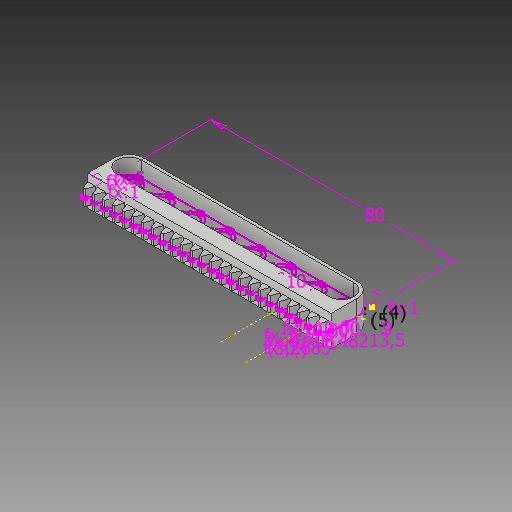
# Autodesk Inventor part: Gear_rack_8
Saved by Autodesk Inventor 2019 (Build 230136000, 136)
## iProperties
Created: 2019-01-28
Part Number: Gear_rack_8
Material: Generic
Document SubType Name: Modeling
Designer: Varga Daniel
Density: 1 g/cm^3
Appearance: Default
Author: Varga Daniel
Autodesk Inventor part; units mm, degrees
ref_plane "YZ Plane" through (0, 0, 0) normal (1, 0, 0) x (0, 1, 0)
ref_plane "XZ Plane" through (0, 0, 0) normal (0, 1, 0) x (-1, 0, 0)
ref_plane "XY Plane" through (0, 0, 0) normal (0, 0, 1) x (1, 0, 0)
derived "Base_part.ipt"
sketch "Sketch1" plane through (0, 0, 0) normal (0, 1, 0) x (-1, 0, 0)
  line L0 (5, 0) -> (25, 0)
  line L1 (30, 5) -> (30, 25)
  line L2 (25, 30) -> (5, 30)
  line L3 (0, 25) -> (0, 5)
  line L4 (5, 29) -> (25, 29)
  line L5 (29, 25) -> (29, 5)
  line L6 (25, 1) -> (5, 1)
  line L7 (1, 5) -> (1, 25)
  circle A0 centre (5, 5) radius 2.5
  circle A1 centre (5, 5) radius 3.5
  arc A2 (25, 0) -> (30, 5) centre (25, 5) ccw
  arc A3 (30, 25) -> (25, 30) centre (25, 25) ccw
  arc A4 (5, 30) -> (0, 25) centre (5, 25) ccw
  arc A5 (0, 5) -> (5, 0) centre (5, 5) ccw
  arc A6 (1, 5) -> (5, 1) centre (5, 5) ccw
  arc A7 (5, 29) -> (1, 25) centre (5, 25) ccw
  arc A8 (29, 25) -> (25, 29) centre (25, 25) ccw
  arc A9 (25, 1) -> (29, 5) centre (25, 5) ccw
  line L8 (49.1041, 15) -> (-27.081, 15) construction
  circle A10 centre (15, 5) radius 2.5
  circle A11 centre (15, 5) radius 3.5
  line L9 (31.1478, 10) -> (-2.4877, 10) construction
  line L10 (-2.8604, 5) -> (35.495, 5) construction
  line L11 (11.5359, 5.5) -> (8.4641, 5.5)
  line L12 (11.5359, 4.5) -> (8.4641, 4.5)
  line L13 (5, -2.5736) -> (5, 36.7522) construction
  line L14 (5.5, 1.5359) -> (5.5, 1)
  line L15 (4.5, 1.5359) -> (4.5, 1.0314)
  line L16 (28.9686, 4.5) -> (1.0314, 4.5)
  line L17 (29, 5.5) -> (1, 5.5)
  line L18 (15, -1.4978) -> (15, 34.8784) construction
  line L19 (15.5, 1.5359) -> (15.5, 1)
  line L20 (14.5, 1.5359) -> (14.5, 1)
  line L21 (1.5359, 5.5) -> (1, 5.5)
  line L22 (1.5359, 4.5) -> (1.0314, 4.5)
  line L23 (28.9686, 4.5) -> (8.4641, 4.5)
  line L24 (29, 5.5) -> (8.4641, 5.5)
  line L25 (4.5, 1.5359) -> (4.5, 1.0314)
  line L26 (5.5, 1.5359) -> (5.5, 1)
  line L27 (29, 10.5) -> (1, 10.5)
  line L28 (29, 9.5) -> (1, 9.5)
  line L29 (4.5, 28.9686) -> (4.5, 10.5)
  line L30 (4.5, 9.5) -> (4.5, 8.4641)
  line L31 (5.5, 29) -> (5.5, 10.5)
  line L32 (5.5, 9.5) -> (5.5, 8.4641)
  point P0 (0, 0)
  point P1 (30, 30)
  point P2 (0, 30)
  point P3 (5, 25)
sketch "Sketch2" plane through (0, 0, 0) normal (0, 1, 0) x (-1, 0, 0)
  circle A0 centre (15, 5) radius 3.5 construction
  circle A1 centre (15, 5) radius 2.5 construction
  line L0 (15.5, 1.5359) -> (15.5, 1) construction
  line L1 (14.5, 1.5359) -> (14.5, 1) construction
  line L2 (25, 1) -> (5, 1) construction
  line L3 (5, 0) -> (25, 0) construction
  arc A2 (0, 5) -> (5, 0) centre (5, 5) ccw construction
  arc A3 (1, 5) -> (5, 1) centre (5, 5) ccw construction
  circle A4 centre (5, 5) radius 3.5 construction
  circle A5 centre (5, 5) radius 2.5 construction
  line L4 (5, -2.5736) -> (5, 36.7522) construction
  line L5 (-2.8604, 5) -> (35.495, 5) construction
  line L6 (29, 5.5) -> (1, 5.5) construction
  line L7 (11.5359, 5.5) -> (8.4641, 5.5) construction
  line L8 (11.5359, 4.5) -> (8.4641, 4.5) construction
  line L9 (5.5, 1.5359) -> (5.5, 1) construction
  line L10 (4.5, 1.5359) -> (4.5, 1.0314) construction
  line L11 (28.9686, 4.5) -> (1.0314, 4.5) construction
  line L12 (15, -1.4978) -> (15, 34.8784) construction
  line L13 (1, 9) -> (1, 5)
  line L14 (0, 13.5) -> (0, 5)
  line L15 (80, 13.5) -> (80, 5)
  line L16 (79, 9) -> (79, 5)
  arc A6 (75, 0) -> (80, 5) centre (75, 5) ccw
  arc A7 (75, 1) -> (79, 5) centre (75, 5) ccw
  arc A8 (1, 5) -> (5, 1) centre (5, 5) ccw
  arc A9 (0, 5) -> (5, 0) centre (5, 5) ccw
  line L17 (5, 0) -> (75, 0)
  circle A10 centre (5, 5) radius 2.5
  arc A11 (8.4641, 4.5) -> (8.4641, 5.5) centre (5, 5) ccw
  arc A12 (12.5, 5) -> (15, 7.5) centre (15, 5) ccw
  circle A13 centre (15, 5) radius 3.5
  line L18 (0, 13.5) -> (80, 13.5)
  line L19 (4.5, 8.4641) -> (4.5, 9)
  line L20 (5.5, 8.4641) -> (5.5, 9)
  line L21 (0.685, 13.5) -> (1.5885, 15.9823)
  line L22 (1.5885, 15.9823) -> (2.2965, 15.9823)
  line L23 (2.2965, 15.9823) -> (3.2, 13.5)
  line L24 (0.685, 13.5) -> (3.2, 13.5)
  line L25 (3.885, 13.5) -> (6.4, 13.5)
  line L26 (3.885, 13.5) -> (4.7885, 15.9823)
  line L27 (4.7885, 15.9823) -> (5.4965, 15.9823)
  line L28 (5.4965, 15.9823) -> (6.4, 13.5)
  line L29 (7.085, 13.5) -> (9.6, 13.5)
  line L30 (7.085, 13.5) -> (7.9885, 15.9823)
  line L31 (7.9885, 15.9823) -> (8.6965, 15.9823)
  line L32 (8.6965, 15.9823) -> (9.6, 13.5)
  line L33 (10.285, 13.5) -> (12.8, 13.5)
  line L34 (10.285, 13.5) -> (11.1885, 15.9823)
  line L35 (11.1885, 15.9823) -> (11.8965, 15.9823)
  line L36 (11.8965, 15.9823) -> (12.8, 13.5)
  line L37 (13.485, 13.5) -> (16, 13.5)
  line L38 (13.485, 13.5) -> (14.3885, 15.9823)
  line L39 (14.3885, 15.9823) -> (15.0965, 15.9823)
  line L40 (15.0965, 15.9823) -> (16, 13.5)
  line L41 (16.685, 13.5) -> (19.2, 13.5)
  line L42 (16.685, 13.5) -> (17.5885, 15.9823)
  line L43 (17.5885, 15.9823) -> (18.2965, 15.9823)
  line L44 (18.2965, 15.9823) -> (19.2, 13.5)
  line L45 (19.885, 13.5) -> (22.4, 13.5)
  line L46 (19.885, 13.5) -> (20.7885, 15.9823)
  line L47 (20.7885, 15.9823) -> (21.4965, 15.9823)
  line L48 (21.4965, 15.9823) -> (22.4, 13.5)
  line L49 (23.085, 13.5) -> (25.6, 13.5)
  line L50 (23.085, 13.5) -> (23.9885, 15.9823)
  line L51 (23.9885, 15.9823) -> (24.6965, 15.9823)
  line L52 (24.6965, 15.9823) -> (25.6, 13.5)
  line L53 (26.285, 13.5) -> (28.8, 13.5)
  line L54 (26.285, 13.5) -> (27.1885, 15.9823)
  line L55 (27.1885, 15.9823) -> (27.8965, 15.9823)
  line L56 (27.8965, 15.9823) -> (28.8, 13.5)
  line L57 (29.485, 13.5) -> (32, 13.5)
  line L58 (29.485, 13.5) -> (30.3885, 15.9823)
  line L59 (30.3885, 15.9823) -> (31.0965, 15.9823)
  line L60 (31.0965, 15.9823) -> (32, 13.5)
  line L61 (32.685, 13.5) -> (35.2, 13.5)
  line L62 (32.685, 13.5) -> (33.5885, 15.9823)
  line L63 (33.5885, 15.9823) -> (34.2965, 15.9823)
  line L64 (34.2965, 15.9823) -> (35.2, 13.5)
  line L65 (35.885, 13.5) -> (38.4, 13.5)
  line L66 (35.885, 13.5) -> (36.7885, 15.9823)
  line L67 (36.7885, 15.9823) -> (37.4965, 15.9823)
  line L68 (37.4965, 15.9823) -> (38.4, 13.5)
  line L69 (39.085, 13.5) -> (41.6, 13.5)
  line L70 (39.085, 13.5) -> (39.9885, 15.9823)
  line L71 (39.9885, 15.9823) -> (40.6965, 15.9823)
  line L72 (40.6965, 15.9823) -> (41.6, 13.5)
  line L73 (42.285, 13.5) -> (44.8, 13.5)
  line L74 (42.285, 13.5) -> (43.1885, 15.9823)
  line L75 (43.1885, 15.9823) -> (43.8965, 15.9823)
  line L76 (43.8965, 15.9823) -> (44.8, 13.5)
  line L77 (45.485, 13.5) -> (48, 13.5)
  line L78 (45.485, 13.5) -> (46.3885, 15.9823)
  line L79 (46.3885, 15.9823) -> (47.0965, 15.9823)
  line L80 (47.0965, 15.9823) -> (48, 13.5)
  line L81 (48.685, 13.5) -> (51.2, 13.5)
  line L82 (48.685, 13.5) -> (49.5885, 15.9823)
  line L83 (49.5885, 15.9823) -> (50.2965, 15.9823)
  line L84 (50.2965, 15.9823) -> (51.2, 13.5)
  line L85 (51.885, 13.5) -> (54.4, 13.5)
  line L86 (51.885, 13.5) -> (52.7885, 15.9823)
  line L87 (52.7885, 15.9823) -> (53.4965, 15.9823)
  line L88 (53.4965, 15.9823) -> (54.4, 13.5)
  line L89 (55.085, 13.5) -> (57.6, 13.5)
  line L90 (55.085, 13.5) -> (55.9885, 15.9823)
  line L91 (55.9885, 15.9823) -> (56.6965, 15.9823)
  line L92 (56.6965, 15.9823) -> (57.6, 13.5)
  line L93 (58.285, 13.5) -> (60.8, 13.5)
  line L94 (58.285, 13.5) -> (59.1885, 15.9823)
  line L95 (59.1885, 15.9823) -> (59.8965, 15.9823)
  line L96 (59.8965, 15.9823) -> (60.8, 13.5)
  line L97 (61.485, 13.5) -> (64, 13.5)
  line L98 (61.485, 13.5) -> (62.3885, 15.9823)
  line L99 (62.3885, 15.9823) -> (63.0965, 15.9823)
  line L100 (63.0965, 15.9823) -> (64, 13.5)
  line L101 (64.685, 13.5) -> (67.2, 13.5)
  line L102 (64.685, 13.5) -> (65.5885, 15.9823)
  line L103 (65.5885, 15.9823) -> (66.2965, 15.9823)
  line L104 (66.2965, 15.9823) -> (67.2, 13.5)
  line L105 (67.885, 13.5) -> (70.4, 13.5)
  line L106 (67.885, 13.5) -> (68.7885, 15.9823)
  line L107 (68.7885, 15.9823) -> (69.4965, 15.9823)
  line L108 (69.4965, 15.9823) -> (70.4, 13.5)
  line L109 (71.085, 13.5) -> (73.6, 13.5)
  line L110 (71.085, 13.5) -> (71.9885, 15.9823)
  line L111 (71.9885, 15.9823) -> (72.6965, 15.9823)
  line L112 (72.6965, 15.9823) -> (73.6, 13.5)
  line L113 (74.285, 13.5) -> (76.8, 13.5)
  line L114 (74.285, 13.5) -> (75.1885, 15.9823)
  line L115 (75.1885, 15.9823) -> (75.8965, 15.9823)
  line L116 (75.8965, 15.9823) -> (76.8, 13.5)
  line L117 (77.485, 13.5) -> (80, 13.5)
  line L118 (77.485, 13.5) -> (78.3885, 15.9823)
  line L119 (78.3885, 15.9823) -> (79.0965, 15.9823)
  line L120 (79.0965, 15.9823) -> (80, 13.5)
  line L121 (28.9686, 4.5) -> (1.0314, 4.5)
  line L122 (1, 5.5) -> (29, 5.5)
  line L123 (4.5, 1.5359) -> (4.5, 1.0314)
  line L124 (5.5, 1.5359) -> (5.5, 1)
  line L125 (14.5, 9) -> (14.5, 8.4641)
  line L126 (14.5, 1.5359) -> (14.5, 1)
  line L127 (15.5, 9) -> (15.5, 8.4641)
  line L128 (15.5, 1.5359) -> (15.5, 1)
  circle A14 centre (15, 5) radius 2.5
  line L129 (5, 1) -> (75, 1)
  line L130 (4.5, 9) -> (5.5, 9)
  line L131 (14.5, 9) -> (15.5, 9)
  line L132 (14.5, 1) -> (15.5, 1)
  arc A15 (5.5, 1.5359) -> (8.4641, 4.5) centre (5, 5) ccw
  arc A16 (8.4641, 5.5) -> (5.5, 1.5359) centre (5, 5) ccw
  line L133 (0, 9) -> (80, 9)
  line L134 (78.4641, 5.5) -> (79, 5.5)
  line L135 (78.4641, 4.5) -> (78.9686, 4.5)
  arc A17 (22.5, 5) -> (25, 7.5) centre (25, 5) ccw
  circle A18 centre (25, 5) radius 2.5
  circle A19 centre (25, 5) radius 3.5
  arc A20 (32.5, 5) -> (35, 7.5) centre (35, 5) ccw
  circle A21 centre (35, 5) radius 2.5
  circle A22 centre (35, 5) radius 3.5
  arc A23 (42.5, 5) -> (45, 7.5) centre (45, 5) ccw
  circle A24 centre (45, 5) radius 2.5
  circle A25 centre (45, 5) radius 3.5
  arc A26 (52.5, 5) -> (55, 7.5) centre (55, 5) ccw
  circle A27 centre (55, 5) radius 2.5
  circle A28 centre (55, 5) radius 3.5
  arc A29 (62.5, 5) -> (65, 7.5) centre (65, 5) ccw
  circle A30 centre (65, 5) radius 2.5
  circle A31 centre (65, 5) radius 3.5
  arc A32 (72.5, 5) -> (75, 7.5) centre (75, 5) ccw
  circle A33 centre (75, 5) radius 2.5
  circle A34 centre (75, 5) radius 3.5
  line L136 (18.4641, 5.5) -> (21.5359, 5.5)
  line L137 (8.4641, 5.5) -> (11.5359, 5.5)
  line L138 (28.4641, 5.5) -> (31.5359, 5.5)
  line L139 (38.4641, 5.5) -> (41.5359, 5.5)
  line L140 (48.4641, 5.5) -> (51.5359, 5.5)
  line L141 (58.4641, 5.5) -> (61.5359, 5.5)
  line L142 (68.4641, 5.5) -> (71.5359, 5.5)
  line L143 (68.4641, 4.5) -> (71.5359, 4.5)
  line L144 (58.4641, 4.5) -> (61.5359, 4.5)
  line L145 (48.4641, 4.5) -> (51.5359, 4.5)
  line L146 (38.4641, 4.5) -> (41.5359, 4.5)
  line L147 (28.4641, 4.5) -> (31.5359, 4.5)
  line L148 (8.4641, 4.5) -> (11.5359, 4.5)
  line L149 (18.4641, 4.5) -> (21.5359, 4.5)
  line L150 (44.5, 1) -> (44.5, 1.5359)
  line L151 (44.5, 8.4641) -> (44.5, 9)
  line L152 (45.5, 9) -> (45.5, 8.4641)
  line L153 (45.5, 1.5359) -> (45.5, 1)
  line L154 (75.5, 1.5359) -> (75.5, 1.0314)
  line L155 (74.5, 1.5359) -> (74.5, 1)
  line L156 (75.5, 8.4641) -> (75.5, 9)
  line L157 (74.5, 8.4641) -> (74.5, 9)
  line L158 (65.5, 8.4641) -> (65.5, 9)
  line L159 (64.5, 8.4641) -> (64.5, 9)
  line L160 (64.5, 1.5359) -> (64.5, 1)
  line L161 (65.5, 1.5359) -> (65.5, 1)
  line L162 (55.5, 8.4641) -> (55.5, 9)
  line L163 (54.5, 8.4641) -> (54.5, 9)
  line L164 (55.5, 1.5359) -> (55.5, 1)
  line L165 (54.5, 1.5359) -> (54.5, 1)
  line L166 (35.5, 8.4641) -> (35.5, 9)
  line L167 (34.5, 8.4641) -> (34.5, 9)
  line L168 (35.5, 1.5359) -> (35.5, 1)
  line L169 (34.5, 1.5359) -> (34.5, 1)
  line L170 (25.5, 8.4641) -> (25.5, 9)
  line L171 (24.5, 8.4641) -> (24.5, 9)
  line L172 (25.5, 1.5359) -> (25.5, 1)
  line L173 (24.5, 1.5359) -> (24.5, 1)
  point P0 (0, 0)
  dimension "d1" = 1
  dimension "d2" = 5
  dimension "d3" = 4
  dimension "d4" = 1
  dimension "d5" = 80
  dimension "d6" = 5
  dimension "d7" = 4
  dimension "d49" = 13.5
  dimension "d50" = 0.708
  dimension "d51" = 110
  dimension "d52" = 110
  dimension "d53" = 0.685
  dimension "d56" = 2.4823
  dimension "d69" = 3.2
  dimension "d72" = 3.2
  dimension "d100" = 9
  dimension "d120" = 10
  constraints: 320 end point, 43 point on circle, 35 collinear, 20 centre point, 20 vertical, 18 point on line, 17 horizontal, 15 coincident, 5 parallel, 3 concentric, 3 tangent, 2 perpendicular, 394 other
  measures "d1" distance between parallel lines of L14 L13
  measures "d2" radius of A2
  measures "d3" radius of A3
  measures "d4" distance between parallel lines of L16 L15
  measures "d5" distance between parallel lines of L14 L15
  measures "d6" radius of A6
  measures "d7" radius of A7
  measures "d49" distance between parallel lines of L3 L18
  measures "d50" distance of L21.end L22.end
  measures "d51" angle of L21 L22
  measures "d52" angle of L23 L22
  measures "d53" distance from line of L14 L21.start
  measures "d56" distance between parallel lines of L18 L22
  measures "d69" distance from line of L23.end L14
  measures "d72" distance of L23.end L25.end
  measures "d100" distance between parallel lines of L3 L130
  measures "d120" distance of A12.centre A17.centre
extrude "Extrusion5" add sketch "Sketch2" along normal blind 5 contours L13 A8 L129 A7 L16 L133 L15 A6 L17 A9 L14 | L133 L14 L18 L15 L131 L130
extrude "Extrusion6" add sketch "Sketch2" against normal blind 5 contours L13 A8 L129 A7 L16 L133 L15 A6 L17 A9 L14 | L133 L14 L18 L15 L131 L130
extrude "Extrusion7" add sketch "Sketch2" along normal blind 2.5 contours L21 L22 L23 L18 | L26 L27 L28 L18 | L30 L31 L32 L18 | L18 L118 L119 L120 | L34 L35 L36 L18 | L18 L114 L115 L116 | L38 L39 L40 L18 | L18 L110 L111 L112 | L42 L43 L44 L18 | L18 L106 L107 L108 | L46 L47 L48 L18 | L18 L102 L103 L104 | L50 L51 L52 L18 | L18 L98 L99 L100 | L54 L55 L56 L18 | L18 L94 L95 L96 | L58 L59 L60 L18 | L18 L90 L91 L92 | L62 L63 L64 L18 | L18 L86 L87 L88 | L66 L67 L68 L18 | L18 L82 L83 L84 | L70 L71 L72 L18 | L18 L78 L79 L80 | L74 L75 L76 L18
extrude "Extrusion8" add sketch "Sketch2" against normal blind 2.5 contours L21 L22 L23 L18 | L26 L27 L28 L18 | L30 L31 L32 L18 | L18 L118 L119 L120 | L34 L35 L36 L18 | L18 L114 L115 L116 | L38 L39 L40 L18 | L18 L110 L111 L112 | L42 L43 L44 L18 | L18 L106 L107 L108 | L46 L47 L48 L18 | L18 L102 L103 L104 | L50 L51 L52 L18 | L18 L98 L99 L100 | L54 L55 L56 L18 | L18 L94 L95 L96 | L58 L59 L60 L18 | L18 L90 L91 L92 | L62 L63 L64 L18 | L18 L86 L87 L88 | L66 L67 L68 L18 | L18 L82 L83 L84 | L70 L71 L72 L18 | L18 L78 L79 L80 | L74 L75 L76 L18
extrude "Extrusion10" [suppressed]
extrude "Extrusion11" [suppressed]
extrude "Extrusion12" [suppressed]
extrude "Extrusion13" [suppressed]
fillet "Fillet1" radius 4 2 edges at (-1, 0, 9) (-79, 0, 9)
equation "\"d1\" = Wall_thickness"
equation "\"d4\" = Wall_thickness"
equation "\"d6\" = d2"
equation "\"d7\" = d3"
equation "\"d52\" = d51"
equation "\"Tooth_error_corrector\" = 0.029"
equation "\"Gear_thickness\" = 5"
equation "\"Wall_thickness\" = 1"
body "Solid2"
